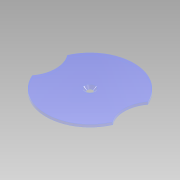
# Autodesk Inventor part: GearCenterCover
Saved by Autodesk Inventor 2021 (Build 250183000, 183)
## iProperties
Created: 2021-05-13
Part Number: GearCenterCover
Material: 一般
Document SubType Name: Modeling
Designer: kumagai
Density: 1 g/cm^3
Appearance: クリア - 青
Author: kumagai
Autodesk Inventor part; units mm, degrees
ref_plane "YZ Plane" through (0, 0, 0) normal (1, 0, 0) x (0, 1, 0)
ref_plane "XZ Plane" through (0, 0, 0) normal (0, 1, 0) x (-1, 0, 0)
ref_plane "XY Plane" through (0, 0, 0) normal (0, 0, 1) x (1, 0, 0)
sketch "スケッチ1" plane through (0, 0, 0) normal (0, 1, 0) x (-1, 0, 0)
  line L0 (0, -24.08) -> (0, 24.08) projected
  line L1 (-51.0552, 0) -> (51.0552, 0) projected
  circle A0 centre (0, 0) radius 17.2
  circle A1 centre (0, 0) radius 1.1
  circle A2 centre (24.968, 0) radius 11.5
  circle A3 centre (-24.968, 0) radius 11.5
  line L2 (1.9153, -7.1479) -> (2.64, -9.8524)
  arc A4 (-1.9153, -7.1479) -> (1.9153, -7.1479) centre (0, 0) ccw
  line L3 (-1.9153, -7.1479) -> (-2.64, -9.8524)
  line L4 (0, -11) -> (0.5714, -10.184)
  line L5 (0, -11) -> (-0.5714, -10.184)
  arc A5 (-2.64, -9.8524) -> (-0.5714, -10.184) centre (0, 0) ccw
  arc A6 (0.5714, -10.184) -> (2.64, -9.8524) centre (0, 0) ccw
  point P0 (-15.76, 6.8893)
  point P1 (-15.76, -6.8893)
  point P2 (15.76, -6.8893)
  point P3 (15.76, 6.8893)
  dimension "d0" = 34.4
  dimension "d1" = 2.2
  dimension "d2" = 24.968
  dimension "d3" = 23
  dimension "d8" = 30
  dimension "d9" = 7.4
  dimension "d11" = 10.2
  dimension "d12" = 11
  dimension "d13" = 70
  constraints: 8 end point, 7 centre point, 6 point on circle, 5 point on line, 4 coincident, 1 concentric, 3 other
  measures "d0" diameter of A0
  measures "d1" diameter of A1
  measures "d2" distance from line of L0 A2.centre
  measures "d3" diameter of A2
  measures "d8" angle of L3 L2
  measures "d9" radius of A4
  measures "d11" radius of A5
  measures "d12" distance from line of L1 L4.start
  measures "d13" angle of L5 L4
extrude "押し出し1" add sketch "スケッチ1" along normal blind 1 contours A0 A3 L1 A1 L0 A4 L3 A5 L5 | L0 L4 A6 L2 A4 A1 L1 A2 A0 | L5 A5 L3 A4 L0 | L0 A4 L2 A6 L4 | A3 A0 L0 A1 L1 | L1 A1 L0 A0 A2
chamfer "面取り1" distance 1 angle 45 1 edges at (1.1, 1, 0)
